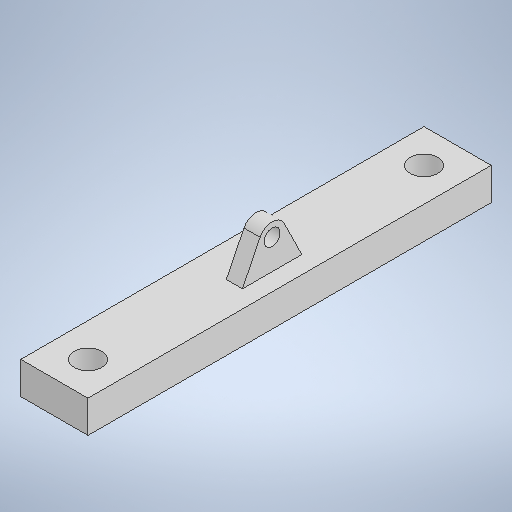
# Autodesk Inventor part: Gripper_arms
Saved by Autodesk Inventor 2025.2 (Build 292293000, 293)
## iProperties
Created: 2025-01-12
Part Number: Gripper_arms
Material: Generic
Document SubType Name: Modeling
Designer: caomi
Density: 1 g/cm^3
Appearance: Default
Author: caomi
Autodesk Inventor part; units mm, degrees
ref_plane "YZ Plane" through (0, 0, 0) normal (1, 0, 0) x (0, 1, 0)
ref_plane "XZ Plane" through (0, 0, 0) normal (0, 1, 0) x (-1, 0, 0)
ref_plane "XY Plane" through (0, 0, 0) normal (0, 0, 1) x (1, 0, 0)
sketch "Sketch1" plane through (0, 0, 0) normal (0, 1, 0) x (-1, 0, 0)
  line L0 (-6.25, 37.5) -> (6.25, 37.5)
  line L1 (6.25, 37.5) -> (6.25, -37.5)
  line L2 (6.25, -37.5) -> (-6.25, -37.5)
  line L3 (-6.25, -37.5) -> (-6.25, 37.5)
  line L4 (-6.25, 37.5) -> (6.25, -37.5) construction
  line L5 (6.25, 37.5) -> (-6.25, -37.5) construction
  circle A0 centre (0, 31.25) radius 2.6
  circle A1 centre (0, -31.25) radius 2.6
  line L6 (13.7936, 0) -> (-15.5073, 0) construction
  point P0 (0, 0)
  dimension "d0" = 5.2
  dimension "d1" = 62.5
  dimension "d2" = 75
  dimension "d3" = 12.5
  constraints: 14 end point, 2 centre point, 2 horizontal, 2 midpoint, 2 parallel, 2 vertical alignment, 1 perpendicular, 1 point on line, 1 other
  measures "d0" diameter of A0
  measures "d1" distance of A0.centre A1.centre
  measures "d2" distance of L0.end L1.end
  measures "d3" distance of L0.start L0.end
extrude "Extrusion1" add sketch "Sketch1" along normal mid plane 6
sketch "Sketch2" plane through (0, 0, 0) normal (1, 0, 0) x (0, 1, 0)
  circle A0 centre (8.5529, 0) radius 2.5
  line L0 (9.6586, -2.2422) -> (2.5464, -5.7497)
  line L1 (3, -37.5) -> (3, 37.5) projected
  line L2 (8.5529, 0) -> (3, 0) construction
  line L3 (9.6586, 2.2422) -> (2.5464, 5.7497)
  circle A1 centre (8.5529, 0) radius 1.5
  point P0 (0, 0)
  point P1 (3, 5.526)
  point P2 (3, -5.526)
  dimension "d6" = 5
  dimension "d7" = 1
  constraints: 6 end point, 2 symmetric about line, 1 centre point, 1 coincident, 1 horizontal alignment, 1 midpoint, 4 other
extrude "Extrusion2" add sketch "Sketch2" along normal blind 3
body "Solid1"
